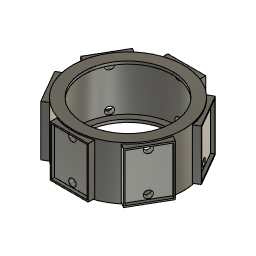
solar_ring (Autodesk Fusion 360 design; units mm, degrees)
Autodesk Fusion 360 part; units mm, degrees
note: some values were not read from the file. Chosen so that the rebuilt part matches the saved one: where a step ends.
sketch "Sketch1" plane through (0, 0, 0) normal (0, 0, 1) x (1, 0, 0)
  circle A0 centre (0, 0) radius 30.125
  circle A1 centre (0, 0) radius 37.625
  dimension "d1" = 60.25
  dimension "d2" = 75.25
  constraint coincident A0.centre A1.centre
  measures "d1" diameter of A0
  measures "d2" diameter of A1
extrude "Extrude1" add sketch "Sketch1" along normal blind 36
sketch "Sketch2" plane through (0, 0, 0) normal (1, 0, 0) x (0, 1, 0)
  line L0 (0, 0) -> (0, 1.85) construction
  line L1 (0, 36) -> (0, 34.15) construction
  line L2 (0, 34.15) -> (0, 1.85)
  line L3 (0, 1.85) -> (34.2775, 1.85)
  line L4 (34.2775, 1.85) -> (34.2775, 34.15)
  line L5 (34.2775, 34.15) -> (0, 34.15)
  dimension "d5" = 1.85
  dimension "d6" = 1.85
  constraint coincident L0.start origin
  constraint vertical L0
  constraint vertical L1
  constraint perpendicular L2 L3
  constraint parallel L2 L4
  constraint parallel L3 L5
  constraint parallel L0 L2
  measures "d5" distance of L0.start L0.end
  measures "d6" distance of L1.start L1.end
revolve "Revolve1" cut sketch "Sketch2" angle 360 about axis through (0, 0, 36) along (0, 0, -1)
ref_plane "WorkPlane1" through (0, 37.625, 23.3376) normal (0, 1, 0) x (1, 0, 0)
sketch "Sketch3" plane through (0, 37.625, 23.3376) normal (0, 1, 0) x (1, 0, 0)
  line L0 (0, 23.3375) -> (0, -12.6625) construction
  line L1 (12.125, 21.5375) -> (-12.125, 21.5375)
  line L2 (-12.125, 21.5375) -> (-12.125, -10.8625)
  line L3 (-12.125, -10.8625) -> (12.125, -10.8625)
  line L4 (12.125, -10.8625) -> (12.125, 21.5375)
  line L5 (12.125, 21.5375) -> (-12.125, -10.8625) construction
  line L6 (-12.125, 21.5375) -> (12.125, -10.8625) construction
  line L7 (-12.8383, -11.8155) -> (12.8383, -11.8155)
  line L8 (12.8383, -11.8155) -> (12.8383, 22.4905)
  line L9 (12.8383, 22.4905) -> (-12.8383, 22.4905)
  line L10 (-12.8383, 22.4905) -> (-12.8383, -11.8155)
  line L11 (-12.8383, -11.8155) -> (12.8383, 22.4905) construction
  line L12 (12.8383, -11.8155) -> (-12.8383, 22.4905) construction
  point P0 (0, 5.3375)
  point P1 (0, 5.3375)
  dimension "d9" = 24.25
  dimension "d10" = 32.4
  constraint vertical L0
  constraint horizontal L1
  constraint perpendicular L1 L2
  constraint parallel L1 L3
  constraint parallel L2 L4
  constraint coincident L5 P1
  constraint coincident L6 P1
  constraint midpoint L0 P1
  constraint horizontal L7
  constraint perpendicular L7 L8
  constraint parallel L7 L9
  constraint parallel L8 L10
  constraint coincident L11 P1
  constraint coincident L12 P1
  constraint coincident P1 P0
  measures "d9" distance of L2.end L3.end
  measures "d10" distance of L1.end L2.end
extrude "Extrude2" add sketch "Sketch3" along normal up to near side of body 1 contours L1 L2 L3 L4
extrude "Extrude3" add sketch "Sketch3" along normal blind 2.15 and the other way up to near side of body 1
sketch "Sketch4" plane through (0, 37.625, 18.0001) normal (0, 1, 0) x (1, 0, 0)
  line L0 (0, -16.2) -> (0, -13.2) construction
  circle A0 centre (0, -13.2) radius 2.5
  line L1 (0, 0) -> (-6, 0) construction
  circle A1 centre (0, 13.2) radius 2.5
  dimension "d17" = 3
  dimension "d18" = 5
  constraint vertical L0
  constraint coincident L0.end A0.centre
  constraint coincident L1.start origin
  constraint horizontal L1
  constraint symmetric A0 L1 A1
  measures "d17" distance of L0.start L0.end
  measures "d18" diameter of A0
extrude "Extrude4" cut sketch "Sketch4" against normal blind 9
pattern_circular "C-Pattern1" count 6 over 360 about axis through (0, 0, 1.75) along (0, 0, 1) of "Extrude2", "Extrude3", "Extrude4"
